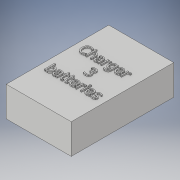
# Autodesk Inventor part: battery charger 2019
Saved by Autodesk Inventor 2019 (Build 230136000, 136)
## iProperties
Created: 2018-12-09
Part Number: battery charger 2019
Material: Generic
Document SubType Name: Modeling
Designer: Tiberus
Density: 1 g/cm^3
Appearance: Default
Author: Tiberus
Autodesk Inventor part; units mm, degrees
ref_plane "YZ Plane" through (0, 0, 0) normal (1, 0, 0) x (0, 1, 0)
ref_plane "XZ Plane" through (0, 0, 0) normal (0, 1, 0) x (-1, 0, 0)
ref_plane "XY Plane" through (0, 0, 0) normal (0, 0, 1) x (1, 0, 0)
sketch "Sketch1" plane through (0, 0, 0) normal (0, 1, 0) x (-1, 0, 0)
  line L0 (0, 0) -> (165.1, 0)
  line L1 (165.1, 0) -> (165.1, -260.35)
  line L2 (165.1, -260.35) -> (0, -260.35)
  line L3 (0, -260.35) -> (0, 0)
  dimension "d0" = 165.1
  dimension "d1" = 260.35
  constraints: 8 end point, 2 parallel, 1 horizontal, 1 perpendicular
  measures "d0" distance of L1.end L2.end
  measures "d1" distance of L0.end L1.end
extrude "Extrusion1" add sketch "Sketch1" along normal blind 76.2
sketch "Sketch2" plane through (0, 76.2, 0) normal (0, 1, 0) x (1, 0, 0)
  line L0 (-163.5139, 239.47) -> (-0.9669, 239.47) construction
  line L1 (-0.9669, 239.47) -> (-0.9669, 25.7814) construction
  line L2 (-0.9669, 25.7814) -> (-163.5139, 25.7814) construction
  line L3 (-163.5139, 25.7814) -> (-163.5139, 239.47) construction
  spline S0 degree 2 poles (-136.0353, 160.9949) (-138.5053, 160.9949) (-142.6838, 162.6621) (-144.207, 164.3294) knots 0 0 0 1 2 2 2
  spline S1 degree 2 poles (-144.207, 164.3294) (-145.7301, 165.9761) (-147.3974, 170.9161) (-147.3974, 174.1271) knots 0 0 0 1 2 2 2
  spline S2 degree 2 poles (-147.3974, 174.1271) (-147.3974, 177.3175) (-145.7713, 182.0517) (-144.2275, 183.8013) knots 0 0 0 1 2 2 2
  spline S3 degree 2 poles (-144.2275, 183.8013) (-142.7044, 185.5098) (-138.5465, 187.3005) (-135.9736, 187.3005) knots 0 0 0 1 2 2 2
  spline S4 degree 2 poles (-135.9736, 187.3005) (-134.6974, 187.3005) (-132.4538, 186.93) (-131.507, 186.6419) knots 0 0 0 1 2 2 2
  spline S5 degree 2 poles (-131.507, 186.6419) (-130.6836, 186.3743) (-128.9752, 185.6127) (-128.1313, 185.1598) knots 0 0 0 1 2 2 2
  line L4 (-128.1313, 185.1598) -> (-128.1313, 181.0843)
  line L5 (-128.1313, 181.0843) -> (-128.3989, 181.0843)
  spline S6 degree 2 poles (-128.3989, 181.0843) (-128.8517, 181.496) (-130.2514, 182.6487) (-131.26, 183.2044) knots 0 0 0 1 2 2 2
  spline S7 degree 2 poles (-131.26, 183.2044) (-132.2274, 183.7396) (-134.5121, 184.4188) (-135.9942, 184.4188) knots 0 0 0 1 2 2 2
  spline S8 degree 2 poles (-135.9942, 184.4188) (-137.6203, 184.4188) (-140.5225, 183.0809) (-141.6134, 181.8047) knots 0 0 0 1 2 2 2
  spline S9 degree 2 poles (-141.6134, 181.8047) (-142.6838, 180.508) (-143.8776, 176.5765) (-143.8776, 174.1271) knots 0 0 0 1 2 2 2
  spline S10 degree 2 poles (-143.8776, 174.1271) (-143.8776, 171.513) (-142.622, 167.7462) (-141.5311, 166.4495) knots 0 0 0 1 2 2 2
  spline S11 degree 2 poles (-141.5311, 166.4495) (-140.4608, 165.1939) (-137.5997, 163.9177) (-135.9942, 163.9177) knots 0 0 0 1 2 2 2
  spline S12 degree 2 poles (-135.9942, 163.9177) (-134.5327, 163.9177) (-132.0421, 164.6381) (-131.0747, 165.1733) knots 0 0 0 1 2 2 2
  spline S13 degree 2 poles (-131.0747, 165.1733) (-130.1485, 165.7085) (-128.7694, 166.82) (-128.3783, 167.2111) knots 0 0 0 1 2 2 2
  line L6 (-128.3783, 167.2111) -> (-128.1313, 167.2111)
  line L7 (-128.1313, 167.2111) -> (-128.1313, 163.1767)
  spline S14 degree 2 poles (-128.1313, 163.1767) (-128.9752, 162.7856) (-130.4572, 162.0652) (-131.507, 161.7359) knots 0 0 0 1 2 2 2
  spline S15 degree 2 poles (-131.507, 161.7359) (-132.6185, 161.3654) (-134.5121, 160.9949) (-136.0353, 160.9949) knots 0 0 0 1 2 2 2
  line L8 (-110.2648, 161.4477) -> (-113.4758, 161.4477)
  line L9 (-113.4758, 161.4477) -> (-113.4758, 172.3158)
  spline S16 degree 2 poles (-113.4758, 172.3158) (-113.4758, 173.6331) (-113.7228, 175.8973) (-114.0933, 176.5765) knots 0 0 0 1 2 2 2
  spline S17 degree 2 poles (-114.0933, 176.5765) (-114.4844, 177.297) (-115.8841, 177.9968) (-117.0779, 177.9968) knots 0 0 0 1 2 2 2
  spline S18 degree 2 poles (-117.0779, 177.9968) (-118.2718, 177.9968) (-120.8036, 176.7206) (-122.018, 175.6914) knots 0 0 0 1 2 2 2
  line L10 (-122.018, 175.6914) -> (-122.018, 161.4477)
  line L11 (-122.018, 161.4477) -> (-125.229, 161.4477)
  line L12 (-125.229, 161.4477) -> (-125.229, 187.9798)
  line L13 (-125.229, 187.9798) -> (-122.018, 187.9798)
  line L14 (-122.018, 187.9798) -> (-122.018, 178.3879)
  spline S19 degree 2 poles (-122.018, 178.3879) (-120.5771, 179.6846) (-117.7984, 181.0432) (-116.234, 181.0432) knots 0 0 0 1 2 2 2
  spline S20 degree 2 poles (-116.234, 181.0432) (-113.4347, 181.0432) (-110.2648, 177.3381) (-110.2648, 173.8184) knots 0 0 0 1 2 2 2
  line L15 (-110.2648, 173.8184) -> (-110.2648, 161.4477)
  spline S21 degree 2 poles (-95.136, 163.4649) (-95.5271, 163.1767) (-96.8444, 162.1475) (-97.4619, 161.8388) knots 0 0 0 1 2 2 2
  spline S22 degree 2 poles (-97.4619, 161.8388) (-98.3058, 161.3859) (-99.8908, 160.9125) (-101.3316, 160.9125) knots 0 0 0 1 2 2 2
  spline S23 degree 2 poles (-101.3316, 160.9125) (-102.5049, 160.9125) (-104.625, 161.7976) (-105.4277, 162.6004) knots 0 0 0 1 2 2 2
  spline S24 degree 2 poles (-105.4277, 162.6004) (-106.1893, 163.3825) (-107.1156, 165.6879) (-107.1156, 166.9641) knots 0 0 0 1 2 2 2
  spline S25 degree 2 poles (-107.1156, 166.9641) (-107.1156, 168.9401) (-105.4483, 171.7394) (-103.6369, 172.5422) knots 0 0 0 1 2 2 2
  spline S26 degree 2 poles (-103.6369, 172.5422) (-102.0314, 173.2832) (-97.6677, 173.8389) (-95.136, 173.983) knots 0 0 0 1 2 2 2
  line L16 (-95.136, 173.983) -> (-95.136, 174.6005)
  spline S27 degree 2 poles (-95.136, 174.6005) (-95.136, 175.712) (-95.8152, 177.0911) (-96.4327, 177.4822) knots 0 0 0 1 2 2 2
  spline S28 degree 2 poles (-96.4327, 177.4822) (-97.0502, 177.8733) (-98.8204, 178.1203) (-99.7673, 178.1203) knots 0 0 0 1 2 2 2
  spline S29 degree 2 poles (-99.7673, 178.1203) (-100.8788, 178.1203) (-103.8839, 177.4616) (-105.3865, 176.8235) knots 0 0 0 1 2 2 2
  line L17 (-105.3865, 176.8235) -> (-105.5718, 176.8235)
  line L18 (-105.5718, 176.8235) -> (-105.5718, 180.0963)
  spline S30 degree 2 poles (-105.5718, 180.0963) (-104.6867, 180.3433) (-101.3728, 180.9608) (-99.7467, 180.9608) knots 0 0 0 1 2 2 2
  spline S31 degree 2 poles (-99.7467, 180.9608) (-97.7707, 180.9608) (-95.0742, 180.3433) (-94.0039, 179.5406) knots 0 0 0 1 2 2 2
  spline S32 degree 2 poles (-94.0039, 179.5406) (-92.9541, 178.7584) (-91.925, 176.2678) (-91.925, 174.477) knots 0 0 0 1 2 2 2
  line L19 (-91.925, 174.477) -> (-91.925, 161.4477)
  line L20 (-91.925, 161.4477) -> (-95.136, 161.4477)
  line L21 (-95.136, 161.4477) -> (-95.136, 163.4649)
  line L22 (-95.136, 166.1407) -> (-95.136, 171.4307)
  spline S33 degree 2 poles (-95.136, 171.4307) (-96.2886, 171.3278) (-99.7673, 170.9778) (-100.8582, 170.6485) knots 0 0 0 1 2 2 2
  spline S34 degree 2 poles (-100.8582, 170.6485) (-102.1344, 170.2574) (-103.8016, 168.6313) (-103.8016, 167.1905) knots 0 0 0 1 2 2 2
  spline S35 degree 2 poles (-103.8016, 167.1905) (-103.8016, 165.5438) (-101.9491, 163.8765) (-100.1789, 163.8765) knots 0 0 0 1 2 2 2
  spline S36 degree 2 poles (-100.1789, 163.8765) (-98.6763, 163.8765) (-96.2063, 165.1733) (-95.136, 166.1407) knots 0 0 0 1 2 2 2
  line L23 (-77.3107, 177.0705) -> (-77.4754, 177.0705)
  spline S37 degree 2 poles (-77.4754, 177.0705) (-77.8459, 177.1735) (-78.6486, 177.2146) (-79.2044, 177.2146) knots 0 0 0 1 2 2 2
  spline S38 degree 2 poles (-79.2044, 177.2146) (-80.5011, 177.2146) (-83.0535, 176.0825) (-84.2062, 174.971) knots 0 0 0 1 2 2 2
  line L24 (-84.2062, 174.971) -> (-84.2062, 161.4477)
  line L25 (-84.2062, 161.4477) -> (-87.4172, 161.4477)
  line L26 (-87.4172, 161.4477) -> (-87.4172, 180.508)
  line L27 (-87.4172, 180.508) -> (-84.2062, 180.508)
  line L28 (-84.2062, 180.508) -> (-84.2062, 177.6675)
  spline S39 degree 2 poles (-84.2062, 177.6675) (-82.4566, 179.2318) (-79.8425, 180.508) (-78.6074, 180.508) knots 0 0 0 1 2 2 2
  spline S40 degree 2 poles (-78.6074, 180.508) (-78.1134, 180.508) (-77.6194, 180.4668) (-77.3107, 180.4051) knots 0 0 0 1 2 2 2
  line L29 (-77.3107, 180.4051) -> (-77.3107, 177.0705)
  spline S41 degree 2 poles (-74.1408, 158.4013) (-73.8115, 158.2573) (-72.5559, 157.8044) (-71.7532, 157.6192) knots 0 0 0 1 2 2 2
  spline S42 degree 2 poles (-71.7532, 157.6192) (-70.8681, 157.3927) (-69.3655, 157.1252) (-68.4804, 157.1252) knots 0 0 0 1 2 2 2
  spline S43 degree 2 poles (-68.4804, 157.1252) (-66.9984, 157.1252) (-64.94, 157.9073) (-64.3637, 158.6072) knots 0 0 0 1 2 2 2
  spline S44 degree 2 poles (-64.3637, 158.6072) (-63.8079, 159.307) (-63.3757, 161.1389) (-63.3757, 162.3122) knots 0 0 0 1 2 2 2
  line L30 (-63.3757, 162.3122) -> (-63.3757, 163.9795)
  spline S45 degree 2 poles (-63.3757, 163.9795) (-64.6724, 162.8474) (-67.163, 161.777) (-69.0361, 161.777) knots 0 0 0 1 2 2 2
  spline S46 degree 2 poles (-69.0361, 161.777) (-72.2883, 161.777) (-76.1374, 166.6141) (-76.1374, 171.1631) knots 0 0 0 1 2 2 2
  spline S47 degree 2 poles (-76.1374, 171.1631) (-76.1374, 173.5302) (-74.7995, 177.194) (-73.688, 178.4908) knots 0 0 0 1 2 2 2
  spline S48 degree 2 poles (-73.688, 178.4908) (-72.6177, 179.7052) (-69.6742, 181.0432) (-68.1099, 181.0432) knots 0 0 0 1 2 2 2
  spline S49 degree 2 poles (-68.1099, 181.0432) (-66.6279, 181.0432) (-64.4666, 180.3433) (-63.3757, 179.7052) knots 0 0 0 1 2 2 2
  line L31 (-63.3757, 179.7052) -> (-63.1904, 180.508)
  line L32 (-63.1904, 180.508) -> (-60.1647, 180.508)
  line L33 (-60.1647, 180.508) -> (-60.1647, 163.6295)
  spline S50 degree 2 poles (-60.1647, 163.6295) (-60.1647, 158.7718) (-64.3843, 154.2435) (-68.7274, 154.2435) knots 0 0 0 1 2 2 2
  spline S51 degree 2 poles (-68.7274, 154.2435) (-70.1271, 154.2435) (-73.0499, 154.6963) (-74.3055, 155.0668) knots 0 0 0 1 2 2 2
  line L34 (-74.3055, 155.0668) -> (-74.3055, 158.4013)
  line L35 (-74.3055, 158.4013) -> (-74.1408, 158.4013)
  line L36 (-63.3757, 166.6141) -> (-63.3757, 177.0911)
  spline S52 degree 2 poles (-63.3757, 177.0911) (-64.5695, 177.6675) (-66.5867, 178.1615) (-67.5953, 178.1615) knots 0 0 0 1 2 2 2
  spline S53 degree 2 poles (-67.5953, 178.1615) (-70.0241, 178.1615) (-72.8235, 174.5799) (-72.8235, 171.2248) knots 0 0 0 1 2 2 2
  spline S54 degree 2 poles (-72.8235, 171.2248) (-72.8235, 168.055) (-70.7034, 164.741) (-68.3157, 164.741) knots 0 0 0 1 2 2 2
  spline S55 degree 2 poles (-68.3157, 164.741) (-67.0601, 164.741) (-64.4254, 165.7291) (-63.3757, 166.6141) knots 0 0 0 1 2 2 2
  spline S56 degree 2 poles (-47.2382, 161.0154) (-51.8078, 161.0154) (-56.8301, 166.1407) (-56.8301, 170.8749) knots 0 0 0 1 2 2 2
  spline S57 degree 2 poles (-56.8301, 170.8749) (-56.8301, 175.5268) (-51.9519, 181.0432) (-48.0204, 181.0432) knots 0 0 0 1 2 2 2
  spline S58 degree 2 poles (-48.0204, 181.0432) (-46.2502, 181.0432) (-43.5126, 180.014) (-42.504, 178.9231) knots 0 0 0 1 2 2 2
  spline S59 degree 2 poles (-42.504, 178.9231) (-41.4749, 177.8321) (-40.3839, 174.6829) (-40.3839, 172.3981) knots 0 0 0 1 2 2 2
  line L37 (-40.3839, 172.3981) -> (-40.3839, 170.6485)
  line L38 (-40.3839, 170.6485) -> (-53.578, 170.6485)
  spline S60 degree 2 poles (-53.578, 170.6485) (-53.578, 167.3346) (-50.2434, 163.8148) (-47.2794, 163.8148) knots 0 0 0 1 2 2 2
  spline S61 degree 2 poles (-47.2794, 163.8148) (-46.2297, 163.8148) (-44.1919, 164.2882) (-43.3686, 164.6587) knots 0 0 0 1 2 2 2
  spline S62 degree 2 poles (-43.3686, 164.6587) (-42.504, 165.0704) (-41.3102, 165.7908) (-40.9191, 166.1201) knots 0 0 0 1 2 2 2
  line L39 (-40.9191, 166.1201) -> (-40.7339, 166.1201)
  line L40 (-40.7339, 166.1201) -> (-40.7339, 162.6209)
  spline S63 degree 2 poles (-40.7339, 162.6209) (-41.2896, 162.3945) (-42.9775, 161.7359) (-43.6361, 161.5506) knots 0 0 0 1 2 2 2
  spline S64 degree 2 poles (-43.6361, 161.5506) (-44.5624, 161.283) (-46.0856, 161.0154) (-47.2382, 161.0154) knots 0 0 0 1 2 2 2
  spline S65 degree 2 poles (-43.5126, 173.0979) (-43.5538, 174.3947) (-44.089, 176.2884) (-44.6036, 176.9265) knots 0 0 0 1 2 2 2
  spline S66 degree 2 poles (-44.6036, 176.9265) (-45.1593, 177.6469) (-46.9089, 178.4085) (-48.2057, 178.4085) knots 0 0 0 1 2 2 2
  spline S67 degree 2 poles (-48.2057, 178.4085) (-49.4818, 178.4085) (-51.2726, 177.6469) (-52.0136, 176.9059) knots 0 0 0 1 2 2 2
  spline S68 degree 2 poles (-52.0136, 176.9059) (-52.734, 176.1443) (-53.475, 174.3124) (-53.578, 173.0979) knots 0 0 0 1 2 2 2
  line L41 (-53.578, 173.0979) -> (-43.5126, 173.0979)
  line L42 (-27.0253, 177.0705) -> (-27.1899, 177.0705)
  spline S69 degree 2 poles (-27.1899, 177.0705) (-27.5604, 177.1735) (-28.3632, 177.2146) (-28.919, 177.2146) knots 0 0 0 1 2 2 2
  spline S70 degree 2 poles (-28.919, 177.2146) (-30.2157, 177.2146) (-32.7681, 176.0825) (-33.9207, 174.971) knots 0 0 0 1 2 2 2
  line L43 (-33.9207, 174.971) -> (-33.9207, 161.4477)
  line L44 (-33.9207, 161.4477) -> (-37.1318, 161.4477)
  line L45 (-37.1318, 161.4477) -> (-37.1318, 180.508)
  line L46 (-37.1318, 180.508) -> (-33.9207, 180.508)
  line L47 (-33.9207, 180.508) -> (-33.9207, 177.6675)
  spline S71 degree 2 poles (-33.9207, 177.6675) (-32.1711, 179.2318) (-29.557, 180.508) (-28.322, 180.508) knots 0 0 0 1 2 2 2
  spline S72 degree 2 poles (-28.322, 180.508) (-27.828, 180.508) (-27.334, 180.4668) (-27.0253, 180.4051) knots 0 0 0 1 2 2 2
  line L48 (-27.0253, 180.4051) -> (-27.0253, 177.0705)
  spline S73 degree 2 poles (-83.0638, 142.619) (-83.99, 142.619) (-85.822, 142.1662) (-86.707, 141.8162) knots 0 0 0 1 2 2 2
  spline S74 degree 2 poles (-86.707, 141.8162) (-87.5304, 141.4663) (-88.7448, 140.7253) (-89.2182, 140.396) knots 0 0 0 1 2 2 2
  line L49 (-89.2182, 140.396) -> (-89.4241, 140.396)
  line L50 (-89.4241, 140.396) -> (-89.4241, 143.9981)
  spline S75 degree 2 poles (-89.4241, 143.9981) (-88.3126, 144.595) (-84.5046, 145.5624) (-82.7962, 145.5624) knots 0 0 0 1 2 2 2
  spline S76 degree 2 poles (-82.7962, 145.5624) (-81.0672, 145.5624) (-78.4942, 144.8626) (-77.4445, 144.1216) knots 0 0 0 1 2 2 2
  spline S77 degree 2 poles (-77.4445, 144.1216) (-76.333, 143.3188) (-75.1803, 140.9929) (-75.1803, 139.4286) knots 0 0 0 1 2 2 2
  spline S78 degree 2 poles (-75.1803, 139.4286) (-75.1803, 137.329) (-77.9385, 134.1592) (-79.8733, 133.7475) knots 0 0 0 1 2 2 2
  line L51 (-79.8733, 133.7475) -> (-79.8733, 133.5005)
  spline S79 degree 2 poles (-79.8733, 133.5005) (-79.0706, 133.3358) (-77.2386, 132.5948) (-76.4565, 131.8538) knots 0 0 0 1 2 2 2
  spline S80 degree 2 poles (-76.4565, 131.8538) (-75.6743, 131.1334) (-74.6863, 128.8281) (-74.6863, 127.1608) knots 0 0 0 1 2 2 2
  spline S81 degree 2 poles (-74.6863, 127.1608) (-74.6863, 125.4524) (-75.8596, 122.5501) (-76.9299, 121.4386) knots 0 0 0 1 2 2 2
  spline S82 degree 2 poles (-76.9299, 121.4386) (-78.0414, 120.2859) (-81.1907, 119.0921) (-83.1873, 119.0921) knots 0 0 0 1 2 2 2
  spline S83 degree 2 poles (-83.1873, 119.0921) (-85.1015, 119.0921) (-88.8477, 120.0183) (-90.1239, 120.6564) knots 0 0 0 1 2 2 2
  line L52 (-90.1239, 120.6564) -> (-90.1239, 124.2585)
  line L53 (-90.1239, 124.2585) -> (-89.8769, 124.2585)
  spline S84 degree 2 poles (-89.8769, 124.2585) (-88.8066, 123.4764) (-85.1839, 122.0355) (-83.3931, 122.0355) knots 0 0 0 1 2 2 2
  spline S85 degree 2 poles (-83.3931, 122.0355) (-82.3433, 122.0355) (-80.2438, 122.6942) (-79.544, 123.4558) knots 0 0 0 1 2 2 2
  spline S86 degree 2 poles (-79.544, 123.4558) (-78.8647, 124.2174) (-78.1443, 126.0287) (-78.1443, 127.4078) knots 0 0 0 1 2 2 2
  spline S87 degree 2 poles (-78.1443, 127.4078) (-78.1443, 128.7869) (-78.9471, 130.5777) (-79.6675, 131.0923) knots 0 0 0 1 2 2 2
  spline S88 degree 2 poles (-79.6675, 131.0923) (-80.3879, 131.6068) (-82.3433, 131.9979) (-83.496, 131.9979) knots 0 0 0 1 2 2 2
  line L54 (-83.496, 131.9979) -> (-84.9369, 131.9979)
  line L55 (-84.9369, 131.9979) -> (-84.9369, 134.8179)
  line L56 (-84.9369, 134.8179) -> (-83.8048, 134.8179)
  spline S89 degree 2 poles (-83.8048, 134.8179) (-81.52, 134.8179) (-78.6383, 136.9997) (-78.6383, 139.0786) knots 0 0 0 1 2 2 2
  spline S90 degree 2 poles (-78.6383, 139.0786) (-78.6383, 140.0461) (-79.3793, 141.4252) (-79.9762, 141.8368) knots 0 0 0 1 2 2 2
  spline S91 degree 2 poles (-79.9762, 141.8368) (-80.6143, 142.2691) (-82.1787, 142.619) (-83.0638, 142.619) knots 0 0 0 1 2 2 2
  spline S92 degree 2 poles (-130.9203, 87.6457) (-130.9203, 82.9733) (-135.4487, 77.2717) (-138.8655, 77.2717) knots 0 0 0 1 2 2 2
  spline S93 degree 2 poles (-138.8655, 77.2717) (-140.4093, 77.2717) (-142.6117, 78.0332) (-143.6821, 78.6919) knots 0 0 0 1 2 2 2
  line L57 (-143.6821, 78.6919) -> (-143.8879, 77.8068)
  line L58 (-143.8879, 77.8068) -> (-146.8931, 77.8068)
  line L59 (-146.8931, 77.8068) -> (-146.8931, 104.3389)
  line L60 (-146.8931, 104.3389) -> (-143.6821, 104.3389)
  line L61 (-143.6821, 104.3389) -> (-143.6821, 94.8705)
  spline S94 degree 2 poles (-143.6821, 94.8705) (-142.4677, 95.9614) (-139.6477, 97.4023) (-137.857, 97.4023) knots 0 0 0 1 2 2 2
  spline S95 degree 2 poles (-137.857, 97.4023) (-134.6254, 97.4023) (-130.9203, 92.2358) (-130.9203, 87.6457) knots 0 0 0 1 2 2 2
  spline S96 degree 2 poles (-134.2343, 87.3987) (-134.2343, 90.8156) (-136.3132, 94.3559) (-138.6185, 94.3559) knots 0 0 0 1 2 2 2
  spline S97 degree 2 poles (-138.6185, 94.3559) (-139.9153, 94.3559) (-142.5912, 93.1209) (-143.6821, 92.1741) knots 0 0 0 1 2 2 2
  line L62 (-143.6821, 92.1741) -> (-143.6821, 81.2443)
  spline S98 degree 2 poles (-143.6821, 81.2443) (-142.4677, 80.6473) (-140.5946, 80.1533) (-139.4831, 80.1533) knots 0 0 0 1 2 2 2
  spline S99 degree 2 poles (-139.4831, 80.1533) (-137.0336, 80.1533) (-134.2343, 83.6319) (-134.2343, 87.3987) knots 0 0 0 1 2 2 2
  spline S100 degree 2 poles (-116.9647, 79.824) (-117.3558, 79.5358) (-118.6732, 78.5067) (-119.2907, 78.1979) knots 0 0 0 1 2 2 2
  spline S101 degree 2 poles (-119.2907, 78.1979) (-120.1346, 77.7451) (-121.7195, 77.2717) (-123.1604, 77.2717) knots 0 0 0 1 2 2 2
  spline S102 degree 2 poles (-123.1604, 77.2717) (-124.3336, 77.2717) (-126.4537, 78.1567) (-127.2565, 78.9595) knots 0 0 0 1 2 2 2
  spline S103 degree 2 poles (-127.2565, 78.9595) (-128.0181, 79.7417) (-128.9443, 82.047) (-128.9443, 83.3232) knots 0 0 0 1 2 2 2
  spline S104 degree 2 poles (-128.9443, 83.3232) (-128.9443, 85.2992) (-127.2771, 88.0986) (-125.4657, 88.9013) knots 0 0 0 1 2 2 2
  spline S105 degree 2 poles (-125.4657, 88.9013) (-123.8602, 89.6423) (-119.4965, 90.1981) (-116.9647, 90.3422) knots 0 0 0 1 2 2 2
  line L63 (-116.9647, 90.3422) -> (-116.9647, 90.9597)
  spline S106 degree 2 poles (-116.9647, 90.9597) (-116.9647, 92.0712) (-117.644, 93.4503) (-118.2615, 93.8413) knots 0 0 0 1 2 2 2
  spline S107 degree 2 poles (-118.2615, 93.8413) (-118.879, 94.2324) (-120.6492, 94.4794) (-121.596, 94.4794) knots 0 0 0 1 2 2 2
  spline S108 degree 2 poles (-121.596, 94.4794) (-122.7075, 94.4794) (-125.7127, 93.8208) (-127.2153, 93.1827) knots 0 0 0 1 2 2 2
  line L64 (-127.2153, 93.1827) -> (-127.4006, 93.1827)
  line L65 (-127.4006, 93.1827) -> (-127.4006, 96.4555)
  spline S109 degree 2 poles (-127.4006, 96.4555) (-126.5155, 96.7025) (-123.2015, 97.32) (-121.5754, 97.32) knots 0 0 0 1 2 2 2
  spline S110 degree 2 poles (-121.5754, 97.32) (-119.5994, 97.32) (-116.903, 96.7025) (-115.8326, 95.8997) knots 0 0 0 1 2 2 2
  spline S111 degree 2 poles (-115.8326, 95.8997) (-114.7829, 95.1175) (-113.7537, 92.6269) (-113.7537, 90.8362) knots 0 0 0 1 2 2 2
  line L66 (-113.7537, 90.8362) -> (-113.7537, 77.8068)
  line L67 (-113.7537, 77.8068) -> (-116.9647, 77.8068)
  line L68 (-116.9647, 77.8068) -> (-116.9647, 79.824)
  line L69 (-116.9647, 82.4999) -> (-116.9647, 87.7898)
  spline S112 degree 2 poles (-116.9647, 87.7898) (-118.1174, 87.6869) (-121.596, 87.337) (-122.6869, 87.0076) knots 0 0 0 1 2 2 2
  spline S113 degree 2 poles (-122.6869, 87.0076) (-123.9631, 86.6166) (-125.6304, 84.9905) (-125.6304, 83.5496) knots 0 0 0 1 2 2 2
  spline S114 degree 2 poles (-125.6304, 83.5496) (-125.6304, 81.9029) (-123.7779, 80.2357) (-122.0077, 80.2357) knots 0 0 0 1 2 2 2
  spline S115 degree 2 poles (-122.0077, 80.2357) (-120.5051, 80.2357) (-118.0351, 81.5324) (-116.9647, 82.4999) knots 0 0 0 1 2 2 2
  spline S116 degree 2 poles (-103.4826, 77.4363) (-106.0967, 77.4363) (-109.0401, 80.4209) (-109.0401, 83.6525) knots 0 0 0 1 2 2 2
  line L70 (-109.0401, 83.6525) -> (-109.0401, 94.2119)
  line L71 (-109.0401, 94.2119) -> (-111.2014, 94.2119)
  line L72 (-111.2014, 94.2119) -> (-111.2014, 96.8671)
  line L73 (-111.2014, 96.8671) -> (-109.0401, 96.8671)
  line L74 (-109.0401, 96.8671) -> (-109.0401, 102.3423)
  line L75 (-109.0401, 102.3423) -> (-105.8291, 102.3423)
  line L76 (-105.8291, 102.3423) -> (-105.8291, 96.8671)
  line L77 (-105.8291, 96.8671) -> (-99.9216, 96.8671)
  line L78 (-99.9216, 96.8671) -> (-99.9216, 94.2119)
  line L79 (-99.9216, 94.2119) -> (-105.8291, 94.2119)
  line L80 (-105.8291, 94.2119) -> (-105.8291, 85.1345)
  spline S117 degree 2 poles (-105.8291, 85.1345) (-105.8291, 83.6937) (-105.7262, 82.1088) (-105.3762, 81.4295) knots 0 0 0 1 2 2 2
  spline S118 degree 2 poles (-105.3762, 81.4295) (-105.0881, 80.8326) (-103.7913, 80.2357) (-102.6798, 80.2357) knots 0 0 0 1 2 2 2
  spline S119 degree 2 poles (-102.6798, 80.2357) (-101.8976, 80.2357) (-100.4362, 80.7091) (-100.1069, 80.8532) knots 0 0 0 1 2 2 2
  line L81 (-100.1069, 80.8532) -> (-99.9216, 80.8532)
  line L82 (-99.9216, 80.8532) -> (-99.9216, 77.9715)
  spline S120 degree 2 poles (-99.9216, 77.9715) (-100.8273, 77.7245) (-102.6798, 77.4363) (-103.4826, 77.4363) knots 0 0 0 1 2 2 2
  spline S121 degree 2 poles (-91.7912, 77.4363) (-94.4053, 77.4363) (-97.3487, 80.4209) (-97.3487, 83.6525) knots 0 0 0 1 2 2 2
  line L83 (-97.3487, 83.6525) -> (-97.3487, 94.2119)
  line L84 (-97.3487, 94.2119) -> (-99.51, 94.2119)
  line L85 (-99.51, 94.2119) -> (-99.51, 96.8671)
  line L86 (-99.51, 96.8671) -> (-97.3487, 96.8671)
  line L87 (-97.3487, 96.8671) -> (-97.3487, 102.3423)
  line L88 (-97.3487, 102.3423) -> (-94.1377, 102.3423)
  line L89 (-94.1377, 102.3423) -> (-94.1377, 96.8671)
  line L90 (-94.1377, 96.8671) -> (-88.2302, 96.8671)
  line L91 (-88.2302, 96.8671) -> (-88.2302, 94.2119)
  line L92 (-88.2302, 94.2119) -> (-94.1377, 94.2119)
  line L93 (-94.1377, 94.2119) -> (-94.1377, 85.1345)
  spline S122 degree 2 poles (-94.1377, 85.1345) (-94.1377, 83.6937) (-94.0348, 82.1088) (-93.6848, 81.4295) knots 0 0 0 1 2 2 2
  spline S123 degree 2 poles (-93.6848, 81.4295) (-93.3967, 80.8326) (-92.0999, 80.2357) (-90.9884, 80.2357) knots 0 0 0 1 2 2 2
  spline S124 degree 2 poles (-90.9884, 80.2357) (-90.2062, 80.2357) (-88.7448, 80.7091) (-88.4155, 80.8532) knots 0 0 0 1 2 2 2
  line L94 (-88.4155, 80.8532) -> (-88.2302, 80.8532)
  line L95 (-88.2302, 80.8532) -> (-88.2302, 77.9715)
  spline S125 degree 2 poles (-88.2302, 77.9715) (-89.1359, 77.7245) (-90.9884, 77.4363) (-91.7912, 77.4363) knots 0 0 0 1 2 2 2
  spline S126 degree 2 poles (-77.5886, 77.3746) (-82.1581, 77.3746) (-87.1805, 82.4999) (-87.1805, 87.2341) knots 0 0 0 1 2 2 2
  spline S127 degree 2 poles (-87.1805, 87.2341) (-87.1805, 91.8859) (-82.3022, 97.4023) (-78.3707, 97.4023) knots 0 0 0 1 2 2 2
  spline S128 degree 2 poles (-78.3707, 97.4023) (-76.6006, 97.4023) (-73.863, 96.3731) (-72.8544, 95.2822) knots 0 0 0 1 2 2 2
  spline S129 degree 2 poles (-72.8544, 95.2822) (-71.8252, 94.1913) (-70.7343, 91.042) (-70.7343, 88.7572) knots 0 0 0 1 2 2 2
  line L96 (-70.7343, 88.7572) -> (-70.7343, 87.0076)
  line L97 (-70.7343, 87.0076) -> (-83.9283, 87.0076)
  spline S130 degree 2 poles (-83.9283, 87.0076) (-83.9283, 83.6937) (-80.5938, 80.1739) (-77.6297, 80.1739) knots 0 0 0 1 2 2 2
  spline S131 degree 2 poles (-77.6297, 80.1739) (-76.58, 80.1739) (-74.5422, 80.6473) (-73.7189, 81.0178) knots 0 0 0 1 2 2 2
  spline S132 degree 2 poles (-73.7189, 81.0178) (-72.8544, 81.4295) (-71.6605, 82.1499) (-71.2694, 82.4793) knots 0 0 0 1 2 2 2
  line L98 (-71.2694, 82.4793) -> (-71.0842, 82.4793)
  line L99 (-71.0842, 82.4793) -> (-71.0842, 78.9801)
  spline S133 degree 2 poles (-71.0842, 78.9801) (-71.6399, 78.7537) (-73.3278, 78.095) (-73.9865, 77.9097) knots 0 0 0 1 2 2 2
  spline S134 degree 2 poles (-73.9865, 77.9097) (-74.9127, 77.6422) (-76.4359, 77.3746) (-77.5886, 77.3746) knots 0 0 0 1 2 2 2
  spline S135 degree 2 poles (-73.863, 89.4571) (-73.9041, 90.7538) (-74.4393, 92.6475) (-74.9539, 93.2856) knots 0 0 0 1 2 2 2
  spline S136 degree 2 poles (-74.9539, 93.2856) (-75.5096, 94.006) (-77.2592, 94.7676) (-78.556, 94.7676) knots 0 0 0 1 2 2 2
  spline S137 degree 2 poles (-78.556, 94.7676) (-79.8322, 94.7676) (-81.6229, 94.006) (-82.3639, 93.265) knots 0 0 0 1 2 2 2
  spline S138 degree 2 poles (-82.3639, 93.265) (-83.0844, 92.5034) (-83.8254, 90.6715) (-83.9283, 89.4571) knots 0 0 0 1 2 2 2
  line L100 (-83.9283, 89.4571) -> (-73.863, 89.4571)
  line L101 (-57.3756, 93.4297) -> (-57.5403, 93.4297)
  spline S139 degree 2 poles (-57.5403, 93.4297) (-57.9108, 93.5326) (-58.7135, 93.5738) (-59.2693, 93.5738) knots 0 0 0 1 2 2 2
  spline S140 degree 2 poles (-59.2693, 93.5738) (-60.566, 93.5738) (-63.1184, 92.4417) (-64.2711, 91.3302) knots 0 0 0 1 2 2 2
  line L102 (-64.2711, 91.3302) -> (-64.2711, 77.8068)
  line L103 (-64.2711, 77.8068) -> (-67.4821, 77.8068)
  line L104 (-67.4821, 77.8068) -> (-67.4821, 96.8671)
  line L105 (-67.4821, 96.8671) -> (-64.2711, 96.8671)
  line L106 (-64.2711, 96.8671) -> (-64.2711, 94.0266)
  spline S141 degree 2 poles (-64.2711, 94.0266) (-62.5215, 95.5909) (-59.9074, 96.8671) (-58.6724, 96.8671) knots 0 0 0 1 2 2 2
  spline S142 degree 2 poles (-58.6724, 96.8671) (-58.1784, 96.8671) (-57.6844, 96.826) (-57.3756, 96.7642) knots 0 0 0 1 2 2 2
  line L107 (-57.3756, 96.7642) -> (-57.3756, 93.4297)
  line L108 (-51.6122, 77.8068) -> (-54.8232, 77.8068)
  line L109 (-54.8232, 77.8068) -> (-54.8232, 96.8671)
  line L110 (-54.8232, 96.8671) -> (-51.6122, 96.8671)
  line L111 (-51.6122, 96.8671) -> (-51.6122, 77.8068)
  line L112 (-51.3858, 100.037) -> (-55.0291, 100.037)
  line L113 (-55.0291, 100.037) -> (-55.0291, 103.3715)
  line L114 (-55.0291, 103.3715) -> (-51.3858, 103.3715)
  line L115 (-51.3858, 103.3715) -> (-51.3858, 100.037)
  spline S143 degree 2 poles (-38.6241, 77.3746) (-43.1936, 77.3746) (-48.216, 82.4999) (-48.216, 87.2341) knots 0 0 0 1 2 2 2
  spline S144 degree 2 poles (-48.216, 87.2341) (-48.216, 91.8859) (-43.3377, 97.4023) (-39.4062, 97.4023) knots 0 0 0 1 2 2 2
  spline S145 degree 2 poles (-39.4062, 97.4023) (-37.6361, 97.4023) (-34.8985, 96.3731) (-33.8899, 95.2822) knots 0 0 0 1 2 2 2
  spline S146 degree 2 poles (-33.8899, 95.2822) (-32.8607, 94.1913) (-31.7698, 91.042) (-31.7698, 88.7572) knots 0 0 0 1 2 2 2
  line L116 (-31.7698, 88.7572) -> (-31.7698, 87.0076)
  line L117 (-31.7698, 87.0076) -> (-44.9638, 87.0076)
  spline S147 degree 2 poles (-44.9638, 87.0076) (-44.9638, 83.6937) (-41.6292, 80.1739) (-38.6652, 80.1739) knots 0 0 0 1 2 2 2
  spline S148 degree 2 poles (-38.6652, 80.1739) (-37.6155, 80.1739) (-35.5777, 80.6473) (-34.7544, 81.0178) knots 0 0 0 1 2 2 2
  spline S149 degree 2 poles (-34.7544, 81.0178) (-33.8899, 81.4295) (-32.696, 82.1499) (-32.3049, 82.4793) knots 0 0 0 1 2 2 2
  line L118 (-32.3049, 82.4793) -> (-32.1197, 82.4793)
  line L119 (-32.1197, 82.4793) -> (-32.1197, 78.9801)
  spline S150 degree 2 poles (-32.1197, 78.9801) (-32.6754, 78.7537) (-34.3633, 78.095) (-35.022, 77.9097) knots 0 0 0 1 2 2 2
  spline S151 degree 2 poles (-35.022, 77.9097) (-35.9482, 77.6422) (-37.4714, 77.3746) (-38.6241, 77.3746) knots 0 0 0 1 2 2 2
  spline S152 degree 2 poles (-34.8985, 89.4571) (-34.9396, 90.7538) (-35.4748, 92.6475) (-35.9894, 93.2856) knots 0 0 0 1 2 2 2
  spline S153 degree 2 poles (-35.9894, 93.2856) (-36.5451, 94.006) (-38.2947, 94.7676) (-39.5915, 94.7676) knots 0 0 0 1 2 2 2
  spline S154 degree 2 poles (-39.5915, 94.7676) (-40.8677, 94.7676) (-42.6584, 94.006) (-43.3994, 93.265) knots 0 0 0 1 2 2 2
  spline S155 degree 2 poles (-43.3994, 93.265) (-44.1198, 92.5034) (-44.8609, 90.6715) (-44.9638, 89.4571) knots 0 0 0 1 2 2 2
  line L120 (-44.9638, 89.4571) -> (-34.8985, 89.4571)
  spline S156 degree 2 poles (-23.3717, 77.354) (-25.286, 77.354) (-28.5999, 78.3832) (-29.6908, 78.9595) knots 0 0 0 1 2 2 2
  line L121 (-29.6908, 78.9595) -> (-29.6908, 82.5616)
  line L122 (-29.6908, 82.5616) -> (-29.5262, 82.5616)
  spline S157 degree 2 poles (-29.5262, 82.5616) (-29.1145, 82.2323) (-28.003, 81.4501) (-27.0767, 81.0178) knots 0 0 0 1 2 2 2
  spline S158 degree 2 poles (-27.0767, 81.0178) (-26.274, 80.6268) (-24.298, 80.0504) (-23.2482, 80.0504) knots 0 0 0 1 2 2 2
  spline S159 degree 2 poles (-23.2482, 80.0504) (-22.4866, 80.0504) (-20.737, 80.4003) (-20.3254, 80.6885) knots 0 0 0 1 2 2 2
  spline S160 degree 2 poles (-20.3254, 80.6885) (-19.7284, 81.0796) (-19.1933, 81.9647) (-19.1933, 82.8704) knots 0 0 0 1 2 2 2
  spline S161 degree 2 poles (-19.1933, 82.8704) (-19.1933, 84.0025) (-20.4283, 85.1757) (-22.0132, 85.5668) knots 0 0 0 1 2 2 2
  spline S162 degree 2 poles (-22.0132, 85.5668) (-22.6307, 85.7109) (-24.6067, 86.1225) (-25.4506, 86.349) knots 0 0 0 1 2 2 2
  spline S163 degree 2 poles (-25.4506, 86.349) (-27.6325, 86.9871) (-29.6085, 89.6217) (-29.6085, 91.4948) knots 0 0 0 1 2 2 2
  spline S164 degree 2 poles (-29.6085, 91.4948) (-29.6085, 94.0884) (-25.7182, 97.32) (-22.5072, 97.32) knots 0 0 0 1 2 2 2
  spline S165 degree 2 poles (-22.5072, 97.32) (-20.9223, 97.32) (-17.7113, 96.5378) (-16.6203, 95.9409) knots 0 0 0 1 2 2 2
  line L123 (-16.6203, 95.9409) -> (-16.6203, 92.5034)
  line L124 (-16.6203, 92.5034) -> (-16.785, 92.5034)
  spline S166 degree 2 poles (-16.785, 92.5034) (-18.02, 93.4914) (-21.0252, 94.6235) (-22.569, 94.6235) knots 0 0 0 1 2 2 2
  spline S167 degree 2 poles (-22.569, 94.6235) (-24.1539, 94.6235) (-26.3357, 93.2856) (-26.3357, 91.9477) knots 0 0 0 1 2 2 2
  spline S168 degree 2 poles (-26.3357, 91.9477) (-26.3357, 90.7332) (-25.039, 89.56) (-23.5981, 89.1895) knots 0 0 0 1 2 2 2
  spline S169 degree 2 poles (-23.5981, 89.1895) (-22.8983, 89.0042) (-21.1281, 88.6337) (-20.1607, 88.4073) knots 0 0 0 1 2 2 2
  spline S170 degree 2 poles (-20.1607, 88.4073) (-18.0612, 87.8721) (-15.9205, 85.4227) (-15.9205, 83.3026) knots 0 0 0 1 2 2 2
  spline S171 degree 2 poles (-15.9205, 83.3026) (-15.9205, 82.0676) (-16.8879, 79.8858) (-17.8348, 79.083) knots 0 0 0 1 2 2 2
  spline S172 degree 2 poles (-17.8348, 79.083) (-18.8433, 78.2391) (-21.4163, 77.354) (-23.3717, 77.354) knots 0 0 0 1 2 2 2
  point P0 (0, 0)
  constraints: 2 other
emboss "Emboss1" sketch "Sketch2" operation add depth 3.175 direction (0, -1, 0)
body "Solid1"
